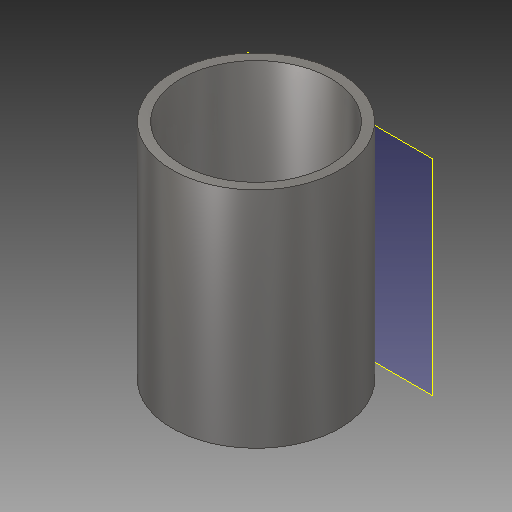
# Autodesk Inventor part: pie
Saved by Autodesk Inventor 2018 (Build 220112000, 112)
## iProperties
Created: 2021-07-05
Part Number: pie
Material: Acero, fundido
Document SubType Name: Modeling
Designer: GABRIEL
Density: 7.85 g/cm^3
Appearance: Semipulido
Author: GABRIEL
Autodesk Inventor part; units mm, degrees
ref_plane "YZ Plane" through (0, 0, 0) normal (1, 0, 0) x (0, 1, 0)
ref_plane "XZ Plane" through (0, 0, 0) normal (0, 1, 0) x (-1, 0, 0)
ref_plane "XY Plane" through (0, 0, 0) normal (0, 0, 1) x (1, 0, 0)
sketch "Boceto1" plane through (0, 0, 0) normal (0, 1, 0) x (-1, 0, 0)
  circle A0 centre (0, 0) radius 40
  circle A1 centre (0, 0) radius 45
  dimension "d0" = 80
  dimension "d1" = 90
  constraints: 2 centre point, 2 coincident
  measures "d0" diameter of A0
  measures "d1" diameter of A1
extrude "Extrusión1" add sketch "Boceto1" along normal blind 120
ref_plane "Plano de trabajo2" through (0, 0, -45) normal (0, 0, -1) x (-1, 0, 0)
ref_plane "Plano de trabajo1" through (-210, 0, -55) normal (0, 0, -1) x (1, 0, 0)
